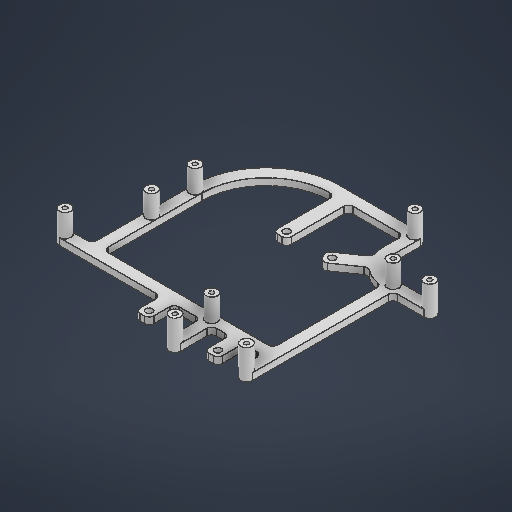
# Autodesk Inventor part: all_pcbs_support
Saved by Autodesk Inventor 2026.1 (Build 301233000, 233)
## iProperties
Created: 2025-11-02
Part Number: all_pcbs_support
Material: Generic
Document SubType Name: Modeling
Designer: emanuel
Density: 1 g/cm^3
Appearance: Default
Author: emanuel
Autodesk Inventor part; units mm, degrees
ref_plane "YZ Plane" through (0, 0, 0) normal (1, 0, 0) x (0, 1, 0)
ref_plane "XZ Plane" through (0, 0, 0) normal (0, 1, 0) x (-1, 0, 0)
ref_plane "XY Plane" through (0, 0, 0) normal (0, 0, 1) x (1, 0, 0)
sketch "Sketch1" plane through (0, 0, 0) normal (0, 1, 0) x (-1, 0, 0)
  circle A0 centre (64, -16) radius 1
  circle A1 centre (0, -16) radius 1
  circle A2 centre (0, 0) radius 1
  circle A3 centre (52.25, -42) radius 1
  circle A4 centre (52.25, -61) radius 1
  circle A5 centre (-12.75, -92) radius 1
  circle A6 centre (-26.75, -4.5) radius 1
  circle A7 centre (-26.75, -68.5) radius 1
  circle A8 centre (-42.75, -68.5) radius 1
  line L0 (-26.75, -4.5) -> (-24.25, -4.5)
  line L1 (-24.25, -4.5) -> (-24.25, -2)
  line L2 (-24.25, -2) -> (-26.75, -2)
  line L3 (-26.75, -2) -> (-26.75, -4.5)
  line L4 (-26.75, -68.5) -> (-29.25, -68.5)
  line L5 (-29.25, -68.5) -> (-29.25, -71)
  line L6 (-29.25, -71) -> (-26.75, -71)
  line L7 (-26.75, -71) -> (-26.75, -68.5)
  line L8 (-42.75, -68.5) -> (-45.25, -68.5)
  line L9 (-45.25, -68.5) -> (-45.25, -66)
  line L10 (-45.25, -66) -> (-42.75, -66)
  line L11 (-42.75, -66) -> (-42.75, -68.5)
  line L12 (-24.25, -2) -> (-29.25, -2)
  line L13 (-29.25, -2) -> (-29.25, -71)
  line L14 (-29.25, -71) -> (-24.25, -71)
  line L15 (-24.25, -71) -> (-24.25, -2)
  line L16 (-24.25, -71) -> (-45.25, -71)
  line L17 (-45.25, -71) -> (-45.25, -66)
  line L18 (-45.25, -66) -> (-24.25, -66)
  line L19 (-24.25, -66) -> (-24.25, -71)
  line L20 (0, 0) -> (2.5, 0)
  line L21 (2.5, 0) -> (2.5, 2.5)
  line L22 (2.5, 2.5) -> (0, 2.5)
  line L23 (0, 2.5) -> (0, 0)
  line L24 (0, -16) -> (-2.5, -16)
  line L25 (-2.5, -16) -> (-2.5, -18.5)
  line L26 (-2.5, -18.5) -> (0, -18.5)
  line L27 (0, -18.5) -> (0, -16)
  line L28 (2.5, 2.5) -> (-2.5, 2.5)
  line L29 (-2.5, 2.5) -> (-2.5, -18.5)
  line L30 (-2.5, -18.5) -> (2.5, -18.5)
  line L31 (2.5, -18.5) -> (2.5, 2.5)
  line L32 (64, -16) -> (66.5, -16)
  line L33 (66.5, -16) -> (66.5, -13.5)
  line L34 (66.5, -13.5) -> (64, -13.5)
  line L35 (64, -13.5) -> (64, -16)
  line L36 (66.5, -13.5) -> (-2.5, -13.5)
  line L37 (-2.5, -13.5) -> (-2.5, -18.5)
  line L38 (-2.5, -18.5) -> (66.5, -18.5)
  line L39 (66.5, -18.5) -> (66.5, -13.5)
  line L40 (52.25, -42) -> (54.75, -42)
  line L41 (54.75, -42) -> (54.75, -39.5)
  line L42 (54.75, -39.5) -> (52.25, -39.5)
  line L43 (52.25, -39.5) -> (52.25, -42)
  line L44 (52.25, -61) -> (49.75, -61)
  line L45 (49.75, -61) -> (49.75, -63.5)
  line L46 (49.75, -63.5) -> (52.25, -63.5)
  line L47 (52.25, -63.5) -> (52.25, -61)
  line L48 (49.75, -63.5) -> (54.75, -63.5)
  line L49 (54.75, -63.5) -> (54.75, -39.5)
  line L50 (54.75, -39.5) -> (49.75, -39.5)
  line L51 (49.75, -39.5) -> (49.75, -63.5)
  line L52 (-12.75, -92) -> (-15.25, -92)
  line L53 (-15.25, -92) -> (-15.25, -94.5)
  line L54 (-15.25, -94.5) -> (-12.75, -94.5)
  line L55 (-12.75, -94.5) -> (-12.75, -92)
  line L56 (-15.25, -94.5) -> (-10.25, -94.5)
  line L57 (-10.25, -94.5) -> (-10.25, -89.5)
  line L58 (-10.25, -89.5) -> (-15.25, -89.5)
  line L59 (-15.25, -89.5) -> (-15.25, -94.5)
  line L60 (49.75, -63.5) -> (-10.25, -63.5)
  line L61 (-10.25, -63.5) -> (-10.25, -89.5)
  line L62 (-10.25, -89.5) -> (49.75, -89.5)
  line L63 (49.75, -89.5) -> (49.75, -63.5)
  line L64 (-10.25, -63.5) -> (54.75, -63.5)
  line L65 (54.75, -63.5) -> (54.75, -94.5)
  line L66 (54.75, -94.5) -> (-10.25, -94.5)
  line L67 (-10.25, -94.5) -> (-10.25, -63.5)
  line L68 (-10.25, -63.5) -> (-15.25, -63.5)
  line L69 (-15.25, -63.5) -> (-15.25, -89.5)
  line L70 (-15.25, -89.5) -> (-10.25, -89.5)
  line L71 (-10.25, -89.5) -> (-10.25, -63.5)
  line L72 (-24.25, -66) -> (-10.25, -66)
  line L73 (-10.25, -66) -> (-10.25, -71)
  line L74 (-10.25, -71) -> (-24.25, -71)
  line L75 (-24.25, -71) -> (-24.25, -66)
  line L76 (49.75, -39.5) -> (54.75, -39.5)
  line L77 (54.75, -39.5) -> (54.75, -18.5)
  line L78 (54.75, -18.5) -> (49.75, -18.5)
  line L79 (49.75, -18.5) -> (49.75, -39.5)
  line L80 (-2.5, -13.5) -> (-24.25, -13.5)
  line L81 (-24.25, -13.5) -> (-24.25, -18.5)
  line L82 (-24.25, -18.5) -> (-2.5, -18.5)
  line L83 (-2.5, -18.5) -> (-2.5, -13.5)
  line L84 (-15.25, -63.5) -> (-10.25, -63.5)
  line L85 (-10.25, -63.5) -> (-10.25, -18.5)
  line L86 (-10.25, -18.5) -> (-15.25, -18.5)
  line L87 (-15.25, -18.5) -> (-15.25, -63.5)
  point P0 (-29.25, -66)
  point P1 (-15.25, -71)
  point P2 (2.5, -13.5)
  point P3 (1, 0)
  point P4 (0, 1)
  dimension "d2" = 2
  dimension "d3" = 2
  dimension "d4" = 2
  dimension "d12" = 2
  dimension "d13" = 2
  dimension "d17" = 2
  dimension "d23" = 2
  dimension "d24" = 2
  dimension "d25" = 2
  dimension "d26" = 2.5
  dimension "d27" = 2.5
  dimension "d28" = 2.5
  dimension "d29" = 2.5
  dimension "d30" = 2.5
  dimension "d31" = 2.5
  dimension "d32" = 2.5
  dimension "d33" = 2.5
  dimension "d34" = 2.5
  dimension "d35" = 2.5
  dimension "d36" = 2.5
  dimension "d37" = 2.5
  dimension "d38" = 2.5
  dimension "d39" = 2.5
  dimension "d40" = 2.5
  dimension "d41" = 2.5
  dimension "d42" = 2.5
  dimension "d43" = 2.5
  dimension "d44" = 5
  dimension "d45" = 5
  constraints: 176 end point, 44 parallel, 22 horizontal, 22 perpendicular, 9 centre point, 7 point on line, 1 coincident
  measures "d2" diameter of A0
  measures "d3" diameter of A1
  measures "d4" diameter of A2
  measures "d12" diameter of A3
  measures "d13" diameter of A4
  measures "d17" diameter of A5
  measures "d23" diameter of A6
  measures "d24" diameter of A7
  measures "d25" diameter of A8
  measures "d26" distance of L2.end L1.end
  measures "d27" distance of L1.end L0.end
  measures "d28" distance of L6.end L5.end
  measures "d29" distance of L5.end L4.end
  measures "d30" distance of L9.end L10.end
  measures "d31" distance of L8.end L9.end
  measures "d32" distance of L22.end L21.end
  measures "d33" distance of L21.end L20.end
  measures "d34" distance of L26.end L25.end
  measures "d35" distance of L25.end L24.end
  measures "d36" distance of L34.end L33.end
  measures "d37" distance of L33.end L32.end
  measures "d38" distance of L42.end L41.end
  measures "d39" distance of L41.end L40.end
  measures "d40" distance of L46.end L45.end
  measures "d41" distance of L45.end L44.end
  measures "d42" distance of L54.end L53.end
  measures "d43" distance of L53.end L52.end
  measures "d44" distance of L58.end L57.end
  measures "d45" distance of L57.end L56.end
extrude "Extrusion1" add sketch "Sketch1" along normal blind 3 contours L32 L39 L38 L31 L36 L35 A0 | A0 L35 L34 L33 L32 | L36 L29 L28 L23 A2 L20 L31 | L31 L30 L27 A1 L24 L29 L36 | L77 L42 L50 L79 L38 | L20 A2 L23 L22 L21 | L29 L25 L82 L15 L80 | L41 L40 A3 L43 L42 | L26 L25 L24 A1 L27 | L15 L18 L13 L12 L3 A6 L0 | L50 L43 A3 L40 L49 L48 L47 A4 L44 L51 | L0 A6 L3 L2 L1 | L44 A4 L47 L46 L45 | L65 L66 L57 L62 L63 L46 L48 | L72 L69 L74 L15 | L15 L14 L7 A7 L4 L13 L18 | L13 L5 L16 L17 L8 A8 L11 L18 | L72 L61 L74 L69 | L56 L55 A5 L52 L59 L58 L57 | L6 L5 L4 A7 L7 | L74 L61 L58 L69 | L11 A8 L8 L9 L10 | L54 L53 L52 A5 L55
fillet "Fillet1" radius 2 9 edges at (2.5, 1.5, -13.5) (24.25, 1.5, -13.5) (-2.5, 1.5, -13.5) (24.25, 1.5, -18.5) (-54.75, 1.5, -18.5) (-49.75, 1.5, -18.5) (29.25, 1.5, -66) (10.25, 1.5, -89.5) (24.25, 1.5, -66)
fillet "Fillet2" radius 10 1 edges at (15.25, 1.5, -71)
fillet "Fillet3" radius 15 1 edges at (10.25, 1.5, -66)
fillet "Fillet4" radius 28 1 edges at (-49.75, 1.5, -89.5)
fillet "Fillet5" radius 32 1 edges at (-54.75, 1.5, -94.5)
sketch "Sketch2" plane through (0, 0, 0) normal (0, -1, 0) x (1, 0, 0)
  line L0 (10.25, -89.5) -> (-19.75, -89.5)
  line L1 (-19.75, -89.5) -> (-19.75, -70.5)
  line L2 (-19.75, -70.5) -> (10.25, -70.5)
  line L3 (10.25, -70.5) -> (10.25, -89.5)
  line L4 (-19.75, -70.5) -> (-36.75, -70.5)
  line L5 (-36.75, -70.5) -> (-36.75, -60.5)
  line L6 (-36.75, -65.5) -> (-26.75, -65.5)
  line L7 (-26.75, -65.5) -> (-16.75, -65.5)
  line L8 (-16.75, -65.5) -> (-6.75, -65.5)
  line L9 (-6.75, -65.5) -> (3.25, -65.5)
  line L10 (3.25, -65.5) -> (13.25, -65.5)
  circle A0 centre (-16.75, -65.5) radius 1.5
  circle A1 centre (3.25, -65.5) radius 1.5
  arc A2 (22.6029, -65.9686) -> (10.25, -80.7332) centre (25.25, -80.7332) ccw projected
  line L11 (3.25, -65.5) -> (25.25, -80.7332)
  line L12 (25.25, -80.7332) -> (26.9578, -78.2668)
  line L13 (26.9578, -78.2668) -> (23.5422, -83.1996)
  line L14 (23.5422, -83.1996) -> (1.5422, -67.9664)
  line L15 (1.5422, -67.9664) -> (3.25, -65.5)
  line L16 (3.25, -65.5) -> (0.7836, -63.7922)
  line L17 (0.7836, -63.7922) -> (-0.9243, -66.2586)
  line L18 (-0.9243, -66.2586) -> (1.5422, -67.9664)
  line L19 (0.7836, -63.7922) -> (2.4914, -61.3257)
  line L20 (2.4914, -61.3257) -> (26.9578, -78.2668)
  line L21 (-16.75, -65.5) -> (-19.75, -65.5)
  line L22 (-19.75, -65.5) -> (-19.75, -62.5)
  line L23 (-19.75, -62.5) -> (-16.75, -62.5)
  line L24 (-16.75, -62.5) -> (-16.75, -65.5)
  line L25 (-19.75, -62.5) -> (-13.75, -62.5)
  line L26 (-13.75, -62.5) -> (-13.75, -89.5)
  line L27 (-13.75, -89.5) -> (-19.75, -89.5)
  line L28 (-19.75, -89.5) -> (-19.75, -62.5)
  line L29 (-16.75, -65.5) -> (-16.75, -5.5)
  line L30 (-16.75, -5.5) -> (13.25, -5.5)
  circle A3 centre (13.25, -5.5) radius 1.5
  circle A4 centre (-16.75, -5.5) radius 1.5
  line L31 (-16.75, -5.5) -> (-13.75, -5.5)
  line L32 (-13.75, -5.5) -> (-13.75, -2.5)
  line L33 (-13.75, -2.5) -> (-16.75, -2.5)
  line L34 (-16.75, -2.5) -> (-16.75, -5.5)
  line L35 (-66.5, -13.5) -> (-4.5, -13.5) projected
  line L36 (-13.75, -2.5) -> (-19.75, -2.5)
  line L37 (-19.75, -2.5) -> (-19.75, -13.5)
  line L38 (-19.75, -13.5) -> (-13.75, -13.5)
  line L39 (-13.75, -13.5) -> (-13.75, -2.5)
  line L40 (13.25, -5.5) -> (16.25, -5.5)
  line L41 (16.25, -5.5) -> (16.25, -2.5)
  line L42 (16.25, -2.5) -> (13.25, -2.5)
  line L43 (13.25, -2.5) -> (13.25, -5.5)
  line L44 (16.25, -2.5) -> (10.25, -2.5)
  line L45 (10.25, -2.5) -> (10.25, -13.5)
  line L46 (10.25, -13.5) -> (16.25, -13.5)
  line L47 (16.25, -13.5) -> (16.25, -2.5)
  point P0 (0, 0)
  point P1 (14.8747, -69.9002)
  point P2 (11.4591, -74.8331)
  dimension "d53" = 19
  dimension "d54" = 17
  dimension "d55" = 10
  dimension "d56" = 10
  dimension "d57" = 10
  dimension "d58" = 10
  dimension "d59" = 10
  dimension "d60" = 10
  dimension "d61" = 3
  dimension "d63" = 3
  dimension "d64" = 3
  dimension "d65" = 6
  dimension "d66" = 3
  dimension "d67" = 3
  dimension "d68" = 3
  dimension "d69" = 3
  dimension "d70" = 6
  dimension "d74" = 60
  dimension "d75" = 30
  dimension "d76" = 3
  dimension "d77" = 3
  dimension "d78" = 3
  dimension "d79" = 3
  dimension "d80" = 6
  dimension "d81" = 3
  dimension "d82" = 3
  constraints: 94 end point, 14 parallel, 13 perpendicular, 11 horizontal, 9 point on line, 4 centre point, 4 coincident, 1 collinear, 1 midpoint, 1 vertical
  measures "d53" distance of L0.end L1.end
  measures "d54" distance of L1.end L4.end
  measures "d55" distance of L4.end L5.end
  measures "d56" distance of L6.start L6.end
  measures "d57" distance of L6.end L7.end
  measures "d58" distance of L7.end L8.end
  measures "d59" distance of L8.end L9.end
  measures "d60" distance of L9.end L10.end
  measures "d61" diameter of A0
  measures "d63" diameter of A1
  measures "d64" distance of L11.end L12.end
  measures "d65" distance of L12.end L13.end
  measures "d66" distance of L11.start L16.end
  measures "d67" distance of L16.end L19.end
  measures "d68" distance of L22.end L23.end
  measures "d69" distance of L21.end L22.end
  measures "d70" distance of L26.end L27.end
  measures "d74" distance of L21.start L29.end
  measures "d75" distance of L29.end L30.end
  measures "d76" diameter of A3
  measures "d77" diameter of A4
  measures "d78" distance of L33.end L32.end
  measures "d79" distance of L32.end L31.end
  measures "d80" distance of L38.end L37.end
  measures "d81" distance of L42.end L41.end
  measures "d82" distance of L41.end L40.end
extrude "Extrusion2" add sketch "Sketch2" against normal blind 3 contours L0 L1 L2 L26 | L2 L28 L7 A0 L8 L26 | L14 L2 L3 | L3 L2 L14 L15 A1 L11 A2 | L8 A0 L24 L25 L26 | L11 A1 L10 L20 A2 | L22 L23 L24 A0 L7 | L18 L17 L9 A1 L15 | L17 L16 A1 L9 | L10 A1 L16 L19 L20 | L35 L37 L36 L34 A4 L29 | L29 A4 L30 L39 L35 | L34 L33 L32 L30 A4 | L45 L44 L43 A3 L30 | L30 A3 L40 L47 L46 L45 | L43 L42 L41 L40 A3
fillet "Fillet6" radius 2 16 edges at (-13.75, 1.5, -62.5) (-19.75, 1.5, -62.5) (2.4914, 1.5, -61.3257) (-0.9243, 1.5, -66.2586) (-13.75, 1.5, -89.5) (14.8747, 1.5, -69.9002) (11.4591, 1.5, -74.8331) (-19.75, 1.5, -13.5) (-13.75, 1.5, -13.5) (-13.75, 1.5, -2.5) (-19.75, 1.5, -2.5) (10.25, 1.5, -13.5) (16.25, 1.5, -13.5) (16.25, 1.5, -2.5) (10.25, 1.5, -2.5) (-19.75, 1.5, -89.5)
fillet "Fillet7" radius 2.5 9 edges at (-66.5, 1.5, -13.5) (-66.5, 1.5, -18.5) (2.5, 1.5, 2.5) (-2.5, 1.5, 2.5) (24.25, 1.5, -2) (29.25, 1.5, -2) (45.25, 1.5, -66) (45.25, 1.5, -71) (15.25, 1.5, -94.5)
sketch "Sketch3" plane through (0, 3, 0) normal (0, 1, 0) x (1, 0, 0)
  circle A0 centre (-52.25, 42) radius 1 projected
  circle A1 centre (-52.25, 42) radius 2.5
  line L0 (-49.75, 20.5) -> (-49.75, 61.5) projected
  circle A2 centre (-52.25, 61) radius 1 projected
  circle A3 centre (-52.25, 61) radius 2.5
  circle A4 centre (12.75, 92) radius 1 projected
  circle A5 centre (12.75, 92) radius 2.5
  line L1 (15.25, 81) -> (15.25, 92) projected
  circle A6 centre (26.75, 68.5) radius 1 projected
  circle A7 centre (26.75, 68.5) radius 2.5
  line L2 (42.75, 71) -> (25.25, 71) projected
  circle A8 centre (42.75, 68.5) radius 1 projected
  circle A9 centre (42.75, 68.5) radius 2.5
  line L3 (45.25, 68) -> (45.25, 69) projected
  circle A10 centre (26.75, 4.5) radius 1 projected
  circle A11 centre (26.75, 4.5) radius 2.5
  circle A12 centre (0, 0) radius 1 projected
  circle A13 centre (0, 0) radius 2.5
  circle A14 centre (-64, 16) radius 1 projected
  circle A15 centre (-64, 16) radius 2.5
  line L4 (-66.5, 16.5) -> (-66.5, 15.5) projected
  circle A16 centre (0, 16) radius 1 projected
  circle A17 centre (0, 16) radius 2.5
  line L5 (22.25, 18.5) -> (-47.75, 18.5) projected
  constraints: 9 centre point, 9 coincident, 7 tangent
extrude "Extrusion3" add sketch "Sketch3" along normal blind 10
body "Solid1"
